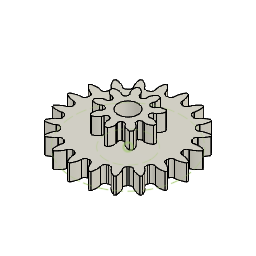
Trasmission-Gear (Autodesk Fusion 360 design; units mm, degrees)
description: Spur Gear; Module: 1.5; Num Teeth: 9; Pressure Angle: 20.0; Backlash: 0.00 mm
description: Spur Gear; Module: 1.65; Num Teeth: 20; Pressure Angle: 20.0; Backlash: 1.00 mm
Autodesk Fusion 360 part; units mm, degrees
sketch "Esboço1" plane through (0, 0, 0) normal (0, 0, 1) x (1, 0, 0) in component "Spur Gear (9 teeth)"
  circle A0 centre (0, 0) radius 4.8992
  circle A1 centre (0, 0) radius 3
  dimension "d20" = 6
  measures "d20" diameter of A1
extrude "Extrusão1" add sketch "Esboço1" along normal blind 5 makes body 1 in component "Spur Gear (9 teeth)"
sketch "Esboço2" plane through (0, 0, 0) normal (0, 0, 1) x (1, 0, 0) in component "Spur Gear (9 teeth)"
  spline S0 degree 5 poles (6.2295, -1.1944) (6.235, -1.1955) (6.2462, -1.1974) (6.263, -1.1997) (6.2856, -1.2016) (6.314, -1.2025) (6.3425, -1.2022) (6.3712, -1.2013) (6.3999, -1.2) (6.4287, -1.1984) (6.4575, -1.1965) (6.4863, -1.1942) (6.5152, -1.1915) (6.5442, -1.1882) (6.5732, -1.1843) (6.6022, -1.1799) (6.6313, -1.1751) (6.6604, -1.1699) (6.6895, -1.1643) (6.7187, -1.1584) (6.7478, -1.1522) (6.777, -1.1457) (6.8062, -1.1388) (6.8354, -1.1315) (6.8646, -1.1239) (6.8938, -1.1159) (6.923, -1.1076) (6.9522, -1.099) (6.9814, -1.0901) (7.0106, -1.0808) (7.0398, -1.0713) (7.069, -1.0614) (7.0982, -1.0513) (7.1274, -1.0408) (7.1565, -1.0301) (7.1857, -1.019) (7.2148, -1.0077) (7.2439, -0.9961) (7.273, -0.9842) (7.302, -0.972) (7.3311, -0.9595) (7.3601, -0.9468) (7.3891, -0.9338) (7.4181, -0.9205) (7.447, -0.9069) (7.4759, -0.8931) (7.5048, -0.879) (7.5336, -0.8647) (7.5624, -0.8501) (7.5911, -0.8352) (7.6199, -0.8201) (7.6485, -0.8047) (7.6772, -0.789) (7.7058, -0.7731) (7.7343, -0.757) (7.7628, -0.7406) (7.7913, -0.7239) (7.8197, -0.707) (7.8481, -0.6899) (7.8764, -0.6725) (7.9046, -0.6549) (7.9328, -0.637) (7.961, -0.6189) (7.989, -0.6006) (8.0171, -0.582) (8.045, -0.5631) (8.073, -0.5441) (8.1008, -0.5248) (8.1286, -0.5053) (8.1563, -0.4855) (8.184, -0.4655) (8.206, -0.4493) (8.2226, -0.4371) (8.2336, -0.4289) (8.2391, -0.4248) knots 0 0 0 0 0 0 0.01428571 0.02857143 0.04285714 0.05714286 0.07142857 0.08571429 0.1 0.11428571 0.12857143 0.14285714 0.15714286 0.17142857 0.18571429 0.2 0.21428571 0.22857143 0.24285714 0.25714286 0.27142857 0.28571429 0.3 0.31428571 0.32857143 0.34285714 0.35714286 0.37142857 0.38571429 0.4 0.41428571 0.42857143 0.44285714 0.45714286 0.47142857 0.48571429 0.5 0.51428571 0.52857143 0.54285714 0.55714286 0.57142857 0.58571429 0.6 0.61428571 0.62857143 0.64285714 0.65714286 0.67142857 0.68571429 0.7 0.71428571 0.72857143 0.74285714 0.75714286 0.77142857 0.78571429 0.8 0.81428571 0.82857143 0.84285714 0.85714286 0.87142857 0.88571429 0.9 0.91428571 0.92857143 0.94285714 0.95714286 0.97142857 0.98571429 1 1 1 1 1 1
  spline S1 degree 5 poles (6.2295, 1.1944) (6.235, 1.1955) (6.2462, 1.1974) (6.263, 1.1997) (6.2856, 1.2016) (6.314, 1.2025) (6.3425, 1.2022) (6.3712, 1.2013) (6.3999, 1.2) (6.4287, 1.1984) (6.4575, 1.1965) (6.4863, 1.1942) (6.5152, 1.1915) (6.5442, 1.1882) (6.5732, 1.1843) (6.6022, 1.1799) (6.6313, 1.1751) (6.6604, 1.1699) (6.6895, 1.1643) (6.7187, 1.1584) (6.7478, 1.1522) (6.777, 1.1457) (6.8062, 1.1388) (6.8354, 1.1315) (6.8646, 1.1239) (6.8938, 1.1159) (6.923, 1.1076) (6.9522, 1.099) (6.9814, 1.0901) (7.0106, 1.0808) (7.0398, 1.0713) (7.069, 1.0614) (7.0982, 1.0513) (7.1274, 1.0408) (7.1565, 1.0301) (7.1857, 1.019) (7.2148, 1.0077) (7.2439, 0.9961) (7.273, 0.9842) (7.302, 0.972) (7.3311, 0.9595) (7.3601, 0.9468) (7.3891, 0.9338) (7.4181, 0.9205) (7.447, 0.9069) (7.4759, 0.8931) (7.5048, 0.879) (7.5336, 0.8647) (7.5624, 0.8501) (7.5911, 0.8352) (7.6199, 0.8201) (7.6485, 0.8047) (7.6772, 0.789) (7.7058, 0.7731) (7.7343, 0.757) (7.7628, 0.7406) (7.7913, 0.7239) (7.8197, 0.707) (7.8481, 0.6899) (7.8764, 0.6725) (7.9046, 0.6549) (7.9328, 0.637) (7.961, 0.6189) (7.989, 0.6006) (8.0171, 0.582) (8.045, 0.5631) (8.073, 0.5441) (8.1008, 0.5248) (8.1286, 0.5053) (8.1563, 0.4855) (8.184, 0.4655) (8.206, 0.4493) (8.2226, 0.4371) (8.2336, 0.4289) (8.2391, 0.4248) knots 0 0 0 0 0 0 0.01428571 0.02857143 0.04285714 0.05714286 0.07142857 0.08571429 0.1 0.11428571 0.12857143 0.14285714 0.15714286 0.17142857 0.18571429 0.2 0.21428571 0.22857143 0.24285714 0.25714286 0.27142857 0.28571429 0.3 0.31428571 0.32857143 0.34285714 0.35714286 0.37142857 0.38571429 0.4 0.41428571 0.42857143 0.44285714 0.45714286 0.47142857 0.48571429 0.5 0.51428571 0.52857143 0.54285714 0.55714286 0.57142857 0.58571429 0.6 0.61428571 0.62857143 0.64285714 0.65714286 0.67142857 0.68571429 0.7 0.71428571 0.72857143 0.74285714 0.75714286 0.77142857 0.78571429 0.8 0.81428571 0.82857143 0.84285714 0.85714286 0.87142857 0.88571429 0.9 0.91428571 0.92857143 0.94285714 0.95714286 0.97142857 0.98571429 1 1 1 1 1 1
  arc A0 (8.2391, -0.4248) -> (8.2391, 0.4248) centre (0, 0) ccw
  line L0 (4.8017, -0.9226) -> (6.2295, -1.1944)
  line L1 (4.8017, 0.9226) -> (6.2295, 1.1944)
  line L2 (4.8017, -0.9226) -> (4.8017, 0.9226)
  point P0 (6.3668, -1.2014)
  point P1 (6.5071, -1.1922)
  point P2 (6.6491, -1.1718)
  point P3 (6.7925, -1.142)
  point P4 (6.9368, -1.1035)
  point P5 (7.0818, -1.0569)
  point P6 (7.2272, -1.0027)
  point P7 (7.3729, -0.941)
  point P8 (7.5185, -0.8722)
  point P9 (7.6639, -0.7963)
  point P10 (7.8088, -0.7135)
  point P11 (7.9531, -0.6239)
  point P12 (8.0966, -0.5276)
  point P13 (6.3668, 1.2014)
  point P14 (6.5071, 1.1922)
  point P15 (6.6491, 1.1718)
  point P16 (6.7925, 1.142)
  point P17 (6.9368, 1.1035)
  point P18 (7.0818, 1.0569)
  point P19 (7.2272, 1.0027)
  point P20 (7.3729, 0.941)
  point P21 (7.5185, 0.8722)
  point P22 (7.6639, 0.7963)
  point P23 (7.8088, 0.7135)
  point P24 (7.9531, 0.6239)
  point P25 (8.0966, 0.5276)
extrude "Extrusão2" add sketch "Esboço2" along normal blind 5 bodies 1 in component "Spur Gear (9 teeth)"
fillet "Arredondamento1" radius 0.88 2 edges at (4.8112, -0.9244, 2.5) (4.8112, 0.9244, 2.5) on bodies 1 in component "Spur Gear (9 teeth)"
pattern_circular "Padrão circular1" count 9 over 360 about axis through (0, 0, 0) along (0, 0, 1) of "Extrusão2", "Arredondamento1" in component "Spur Gear (9 teeth)"
sketch "Esboço3" plane through (0, 0, 0) normal (0, 0, 1) x (1, 0, 0) in component "Spur Gear (9 teeth)"
  circle A0 centre (0, 0) radius 6.75 construction
move_body "Mover1" bodies 1 to x (1, 0, 0) y (0, 1, 0) z (0, 0, 1) at (0, 0, 5) in component "Spur Gear (9 teeth)"
sketch "Esboço1 (2)" plane through (0, 0, 0) normal (0, 0, 1) x (1, 0, 0) in component "Spur Gear (20 teeth)"
  circle A0 centre (0, 0) radius 14.4692
  circle A1 centre (0, 0) radius 3
extrude "Extrusão1'" add sketch "Esboço1 (2)" along normal blind 5 separate body makes body 2 in component "Spur Gear (20 teeth)"
sketch "Esboço2 (2)" plane through (0, 0, 0) normal (0, 0, 1) x (1, 0, 0) in component "Spur Gear (20 teeth)"
  spline S0 degree 5 poles (15.4574, -1.2127) (15.4652, -1.2133) (15.4806, -1.2143) (15.5039, -1.2152) (15.5349, -1.2152) (15.5737, -1.2136) (15.6125, -1.2109) (15.6514, -1.2074) (15.6903, -1.2036) (15.7292, -1.1995) (15.7681, -1.1951) (15.807, -1.1904) (15.8459, -1.1851) (15.8849, -1.1793) (15.9238, -1.173) (15.9627, -1.1661) (16.0017, -1.1588) (16.0406, -1.1511) (16.0795, -1.1431) (16.1184, -1.1348) (16.1573, -1.1261) (16.1962, -1.1171) (16.2351, -1.1078) (16.274, -1.0982) (16.3129, -1.0881) (16.3517, -1.0778) (16.3905, -1.0671) (16.4294, -1.0562) (16.4682, -1.0449) (16.5069, -1.0333) (16.5457, -1.0215) (16.5844, -1.0094) (16.6232, -0.997) (16.6619, -0.9843) (16.7006, -0.9713) (16.7392, -0.9581) (16.7779, -0.9445) (16.8165, -0.9308) (16.8551, -0.9167) (16.8936, -0.9024) (16.9322, -0.8878) (16.9707, -0.873) (17.0092, -0.858) (17.0476, -0.8426) (17.086, -0.8271) (17.1244, -0.8113) (17.1628, -0.7952) (17.2011, -0.7789) (17.2394, -0.7624) (17.2777, -0.7456) (17.3159, -0.7286) (17.3541, -0.7114) (17.3923, -0.6939) (17.4304, -0.6762) (17.4685, -0.6583) (17.5066, -0.6401) (17.5446, -0.6217) (17.5826, -0.6031) (17.6206, -0.5843) (17.6585, -0.5653) (17.6964, -0.546) (17.7342, -0.5265) (17.772, -0.5069) (17.8097, -0.4869) (17.8474, -0.4668) (17.8851, -0.4465) (17.9227, -0.4259) (17.9603, -0.4052) (17.9979, -0.3842) (18.0353, -0.3631) (18.0728, -0.3417) (18.1027, -0.3244) (18.1251, -0.3114) (18.1401, -0.3026) (18.1475, -0.2983) knots 0 0 0 0 0 0 0.01428571 0.02857143 0.04285714 0.05714286 0.07142857 0.08571429 0.1 0.11428571 0.12857143 0.14285714 0.15714286 0.17142857 0.18571429 0.2 0.21428571 0.22857143 0.24285714 0.25714286 0.27142857 0.28571429 0.3 0.31428571 0.32857143 0.34285714 0.35714286 0.37142857 0.38571429 0.4 0.41428571 0.42857143 0.44285714 0.45714286 0.47142857 0.48571429 0.5 0.51428571 0.52857143 0.54285714 0.55714286 0.57142857 0.58571429 0.6 0.61428571 0.62857143 0.64285714 0.65714286 0.67142857 0.68571429 0.7 0.71428571 0.72857143 0.74285714 0.75714286 0.77142857 0.78571429 0.8 0.81428571 0.82857143 0.84285714 0.85714286 0.87142857 0.88571429 0.9 0.91428571 0.92857143 0.94285714 0.95714286 0.97142857 0.98571429 1 1 1 1 1 1
  spline S1 degree 5 poles (15.4574, 1.2127) (15.4652, 1.2133) (15.4806, 1.2143) (15.5039, 1.2152) (15.5349, 1.2152) (15.5737, 1.2136) (15.6125, 1.2109) (15.6514, 1.2074) (15.6903, 1.2036) (15.7292, 1.1995) (15.7681, 1.1951) (15.807, 1.1904) (15.8459, 1.1851) (15.8849, 1.1793) (15.9238, 1.173) (15.9627, 1.1661) (16.0017, 1.1588) (16.0406, 1.1511) (16.0795, 1.1431) (16.1184, 1.1348) (16.1573, 1.1261) (16.1962, 1.1171) (16.2351, 1.1078) (16.274, 1.0982) (16.3129, 1.0881) (16.3517, 1.0778) (16.3905, 1.0671) (16.4294, 1.0562) (16.4682, 1.0449) (16.5069, 1.0333) (16.5457, 1.0215) (16.5844, 1.0094) (16.6232, 0.997) (16.6619, 0.9843) (16.7006, 0.9713) (16.7392, 0.9581) (16.7779, 0.9445) (16.8165, 0.9308) (16.8551, 0.9167) (16.8936, 0.9024) (16.9322, 0.8878) (16.9707, 0.873) (17.0092, 0.858) (17.0476, 0.8426) (17.086, 0.8271) (17.1244, 0.8113) (17.1628, 0.7952) (17.2011, 0.7789) (17.2394, 0.7624) (17.2777, 0.7456) (17.3159, 0.7286) (17.3541, 0.7114) (17.3923, 0.6939) (17.4304, 0.6762) (17.4685, 0.6583) (17.5066, 0.6401) (17.5446, 0.6217) (17.5826, 0.6031) (17.6206, 0.5843) (17.6585, 0.5653) (17.6964, 0.546) (17.7342, 0.5265) (17.772, 0.5069) (17.8097, 0.4869) (17.8474, 0.4668) (17.8851, 0.4465) (17.9227, 0.4259) (17.9603, 0.4052) (17.9979, 0.3842) (18.0353, 0.3631) (18.0728, 0.3417) (18.1027, 0.3244) (18.1251, 0.3114) (18.1401, 0.3026) (18.1475, 0.2983) knots 0 0 0 0 0 0 0.01428571 0.02857143 0.04285714 0.05714286 0.07142857 0.08571429 0.1 0.11428571 0.12857143 0.14285714 0.15714286 0.17142857 0.18571429 0.2 0.21428571 0.22857143 0.24285714 0.25714286 0.27142857 0.28571429 0.3 0.31428571 0.32857143 0.34285714 0.35714286 0.37142857 0.38571429 0.4 0.41428571 0.42857143 0.44285714 0.45714286 0.47142857 0.48571429 0.5 0.51428571 0.52857143 0.54285714 0.55714286 0.57142857 0.58571429 0.6 0.61428571 0.62857143 0.64285714 0.65714286 0.67142857 0.68571429 0.7 0.71428571 0.72857143 0.74285714 0.75714286 0.77142857 0.78571429 0.8 0.81428571 0.82857143 0.84285714 0.85714286 0.87142857 0.88571429 0.9 0.91428571 0.92857143 0.94285714 0.95714286 0.97142857 0.98571429 1 1 1 1 1 1
  arc A0 (18.1475, -0.2983) -> (18.1475, 0.2983) centre (0, 0) ccw
  line L0 (14.4149, -1.1317) -> (15.4574, -1.2127)
  line L1 (14.4149, 1.1317) -> (15.4574, 1.2127)
  line L2 (14.4149, -1.1317) -> (14.4149, 1.1317)
  point P0 (15.6473, -1.2077)
  point P1 (15.8384, -1.186)
  point P2 (16.0303, -1.1531)
  point P3 (16.2227, -1.1108)
  point P4 (16.4154, -1.0601)
  point P5 (16.6084, -1.0017)
  point P6 (16.8014, -0.9361)
  point P7 (16.9945, -0.8637)
  point P8 (17.1874, -0.7847)
  point P9 (17.3802, -0.6994)
  point P10 (17.5727, -0.608)
  point P11 (17.7648, -0.5106)
  point P12 (17.9564, -0.4073)
  point P13 (15.6473, 1.2077)
  point P14 (15.8384, 1.186)
  point P15 (16.0303, 1.1531)
  point P16 (16.2227, 1.1108)
  point P17 (16.4154, 1.0601)
  point P18 (16.6084, 1.0017)
  point P19 (16.8014, 0.9361)
  point P20 (16.9945, 0.8637)
  point P21 (17.1874, 0.7847)
  point P22 (17.3802, 0.6994)
  point P23 (17.5727, 0.608)
  point P24 (17.7648, 0.5106)
  point P25 (17.9564, 0.4073)
extrude "Extrusão2'" add sketch "Esboço2 (2)" along normal blind 5 bodies 2 in component "Spur Gear (20 teeth)"
fillet "Arredondamento1'" radius 0.97 2 edges at (14.4248, -1.1324, 2.5) (14.4248, 1.1324, 2.5) on bodies 2 in component "Spur Gear (20 teeth)"
pattern_circular "Padrão circular1'" count 20 over 360 about axis through (0, 0, 0) along (0, 0, 1) of "Extrusão2'", "Arredondamento1'" in component "Spur Gear (20 teeth)"
sketch "Esboço3 (2)" plane through (0, 0, 0) normal (0, 0, 1) x (1, 0, 0) in component "Spur Gear (20 teeth)"
  circle A0 centre (0, 0) radius 16.5 construction
component "Spur Gear (9 teeth)" placed x (1, 0, 0) y (0, 1, 0) z (0, 0, 1) at (0, 0, 0)
component "Spur Gear (20 teeth)" placed x (1, 0, 0) y (0, 1, 0) z (0, 0, 1) at (0, 0, 0)
